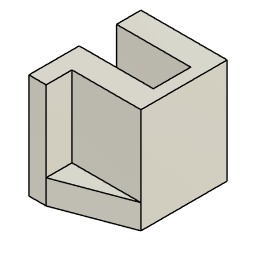
colour_sensor_servo_seat_bottom (Autodesk Fusion 360 design; units mm, degrees)
part number: 2025-09-29-11-37-15-270
part number: 2025-09-29-11-38-54-172
Autodesk Fusion 360 part; units mm, degrees
sketch "Colour Sensor Servo Seat Outline" plane through (0, 0, 0) normal (0, 0, 1) x (1, 0, 0) in component "Colour Sensor Servo Seat Bottom"
  line L0 (0, 0) -> (54.5, 0)
  line L1 (54.5, 0) -> (54.5, 39)
  line L2 (54.5, 39) -> (0, 39)
  line L3 (0, 39) -> (0, 0)
  dimension "d1" = 39
  dimension "d2" = 54.5
  constraint horizontal L0
  constraint vertical L1
  constraint horizontal L2
  constraint vertical L3
  constraint coincident L0.start L3.end
  measures "d1" distance of L0.end L1.end
  measures "d2" distance of L0.start L0.end
extrude "Extrude1" add sketch "Colour Sensor Servo Seat Outline" along normal blind 30 in component "Colour Sensor Servo Seat Bottom"
sketch "Colour Sensor Servo Hole" plane through (0, 0, 30) normal (0, 0, 1) x (-1, 0, 0) in component "Colour Sensor Servo Seat Bottom"
  line L0 (0, -39) -> (0, 0)
  line L1 (0, 0) -> (-54.5, 0)
  line L2 (-54.5, 0) -> (-54.5, -39)
  line L3 (-54.5, -39) -> (0, -39)
  line L4 (-54.5, -8.5) -> (-18, -8.5)
  line L5 (-18, -8.5) -> (-18, -21.5)
  line L6 (-18, -21.5) -> (-54.5, -21.5)
  line L7 (-54.5, -21.5) -> (-54.5, -8.5)
  line L8 (-54.5, 0) -> (-18, 0)
  line L9 (-18, 0) -> (-18, -30)
  line L10 (-18, -30) -> (-54.5, -30)
  line L11 (-54.5, -30) -> (-54.5, 0)
  line L12 (-54.5, -21.5) -> (-49.8, -21.5)
  line L13 (-49.8, -21.5) -> (-49.8, -8.5)
  line L14 (-49.8, -8.5) -> (-54.5, -8.5)
  line L15 (-54.5, -8.5) -> (-54.5, -21.5)
  point P0 (-54.5, -21.5)
  point P1 (-54.5, -30)
  dimension "d6" = 13
  dimension "d8" = 36.5
  dimension "d9" = 30
  dimension "d10" = 8.5
  dimension "d11" = 8.5
  dimension "d12" = 4.7
  constraint horizontal L4
  constraint vertical L5
  constraint horizontal L6
  constraint vertical L7
  constraint coincident L2 L4.start
  constraint horizontal L8
  constraint vertical L9
  constraint horizontal L10
  constraint vertical L11
  constraint coincident L1.end L2.start
  constraint collinear L5 L9
  constraint coincident P0 L6.end
  constraint coincident P1 L10.end
  constraint horizontal L12
  constraint vertical L13
  constraint horizontal L14
  constraint vertical L15
  constraint coincident L4 L13.end
  measures "d6" distance of L4.start P0
  measures "d8" distance of L4.start L4.end
  measures "d9" distance of L1.end P1
  measures "d10" distance of L6 L10
  measures "d11" distance of L4 L8
  measures "d12" distance of L11 L13
extrude "Extrude2" cut sketch "Colour Sensor Servo Hole" against normal blind 5 contours L2 L4 L6 L7 L11 L12 L13 L14 L15 in component "Colour Sensor Servo Seat Bottom"
extrude "Extrude3" cut sketch "Colour Sensor Servo Hole" against normal blind 25.82 contours L4 L5 L6 L9 L13 in component "Colour Sensor Servo Seat Bottom"
chamfer "Chamfer1" distance 24 distance2 9 1 edges at (27.25, 39, 0) measured on face at (36.3333, 39, 20) in component "Colour Sensor Servo Seat Bottom"
sketch "Front Ribs" plane through (0, 39, 0) normal (0, 1, 0) x (-1, 0, 0) in component "Colour Sensor Servo Seat Bottom"
  line L0 (-54.5, 24) -> (0, 24)
  line L1 (0, 24) -> (0, 30)
  line L2 (0, 30) -> (-54.5, 30)
  line L3 (-54.5, 30) -> (-54.5, 24)
  line L4 (0, 0) -> (0, 24)
  line L5 (0, 24) -> (-54.5, 24)
  line L6 (-54.5, 24) -> (-54.5, 0)
  line L7 (-54.5, 0) -> (0, 0)
  line L8 (-46, 24) -> (-18, 24)
  line L9 (-18, 24) -> (-18, 0)
  line L10 (-18, 0) -> (-46, 0)
  line L11 (-46, 0) -> (-46, 24)
  line L12 (-18, 24) -> (-9.5, 24)
  line L13 (-9.5, 24) -> (-9.5, 0)
  line L14 (-9.5, 0) -> (-18, 0)
  line L15 (-18, 0) -> (-18, 24)
  dimension "d26" = 8.5
  dimension "d31" = 8.5
  dimension "d39" = 9.5
  constraint horizontal L8
  constraint vertical L9
  constraint horizontal L10
  constraint vertical L11
  constraint coincident L7 L9.end
  constraint coincident L0 L8.start
  constraint horizontal L12
  constraint vertical L13
  constraint horizontal L14
  constraint vertical L15
  constraint coincident L7 L13.end
  measures "d26" distance of L6 L11
  measures "d31" distance of L13 L15
  measures "d39" distance of L4 L13
extrude "Extrude4" cut sketch "Front Ribs" against normal blind 9 contours L0 L5 L7 L8 L9 L10 L11 L15 | L0 L4 L5 L7 L13 in component "Colour Sensor Servo Seat Bottom"
chamfer "Chamfer2" distance 24 distance2 9.5 1 edges at (0, 15, 0) measured on face at (0, 10, 18) in component "Colour Sensor Servo Seat Bottom"
sketch "Side Ribs" plane through (0, 0, 0) normal (-1, 0, 0) x (0, -1, 0) in component "Colour Sensor Servo Seat Bottom"
  line L0 (-30, 24) -> (0, 24)
  line L1 (0, 24) -> (0, 30)
  line L2 (0, 30) -> (-39, 30)
  line L3 (-39, 30) -> (-39, 24)
  line L4 (-39, 24) -> (-30, 24)
  line L5 (0, 0) -> (0, 24)
  line L6 (0, 24) -> (-30, 24)
  line L7 (-30, 24) -> (-30, 0)
  line L8 (-30, 0) -> (0, 0)
  line L9 (-21.5, 24) -> (-8.5, 24)
  line L10 (-8.5, 24) -> (-8.5, 0)
  line L11 (-8.5, 0) -> (-21.5, 0)
  line L12 (-21.5, 0) -> (-21.5, 24)
  dimension "d33" = 8.5
  dimension "d34" = 8.5
  constraint horizontal L9
  constraint vertical L10
  constraint horizontal L11
  constraint vertical L12
  constraint coincident L8 L10.end
  constraint coincident L0 L9.start
  measures "d33" distance of L7 L12
  measures "d34" distance of L5 L10
extrude "Extrude6" cut sketch "Side Ribs" against normal blind 9.5 contours L0 L6 L8 L9 L10 L11 L12 in component "Colour Sensor Servo Seat Bottom"
chamfer "Chamfer3" distance 9.5 distance2 9 1 edges at (0, 39, 27) measured on face at (24.1667, 39, 28) in component "Colour Sensor Servo Seat Bottom"
sketch "Servo Cable Hole" plane through (9.5, 0, 0) normal (-1, 0, 0) x (0, -1, 0) in component "Colour Sensor Servo Seat Bottom"
  line L0 (-21.5, 0) -> (-8.5, 0)
  line L1 (-8.5, 0) -> (-8.5, 24)
  line L2 (-8.5, 24) -> (-21.5, 24)
  line L3 (-21.5, 24) -> (-21.5, 0)
  line L4 (-21.5, 0) -> (-21.5, 24)
  line L5 (-21.5, 24) -> (-30, 24)
  line L6 (-30, 24) -> (-30, 0)
  line L7 (-30, 0) -> (-21.5, 0)
  line L8 (-8.5, 24) -> (-8.5, 0)
  line L9 (-8.5, 0) -> (0, 0)
  line L10 (0, 0) -> (0, 24)
  line L11 (0, 24) -> (-8.5, 24)
  line L12 (-21.5, 14.18) -> (-8.5, 14.18)
  line L13 (-8.5, 14.18) -> (-8.5, 4.18)
  line L14 (-8.5, 4.18) -> (-21.5, 4.18)
  line L15 (-21.5, 4.18) -> (-21.5, 14.18)
  dimension "d40" = 10
  dimension "d41" = 4.18
  constraint horizontal L12
  constraint vertical L13
  constraint horizontal L14
  constraint vertical L15
  constraint coincident L4 L12.start
  measures "d40" distance of L12.start L14.end
  measures "d41" distance of L0 L14
extrude "Extrude7" cut sketch "Servo Cable Hole" against normal blind 8.5 contours L1 L3 L4 L8 L12 L13 L14 L15 in component "Colour Sensor Servo Seat Bottom"
sketch "Top Segment" plane through (0, 0, 0) normal (0, -1, 0) x (1, 0, 0)
  line L0 (6, 45) -> (0, 45)
  line L1 (0, 45) -> (0, 0)
  line L2 (0, 0) -> (6, 0)
  line L3 (6, 0) -> (6, 8.5)
  line L4 (6, 8.5) -> (6, 36.5)
  line L5 (6, 36.5) -> (6, 45)
  line L6 (30, 8.5) -> (6, 8.5)
  line L7 (6, 8.5) -> (6, 0)
  line L8 (6, 0) -> (30, 0)
  line L9 (30, 0) -> (30, 8.5)
  line L10 (0, 54.5) -> (0, 45)
  line L11 (0, 45) -> (6, 45)
  line L12 (6, 45) -> (6, 54.5)
  line L13 (6, 54.5) -> (0, 54.5)
  line L14 (30, 45) -> (6, 54.5)
  line L15 (6, 54.5) -> (6, 45)
  line L16 (6, 45) -> (30, 45)
  line L17 (6, 36.5) -> (30, 36.5)
  line L18 (30, 36.5) -> (30, 45)
  line L19 (30, 45) -> (6, 45)
  line L20 (6, 45) -> (6, 36.5)
  line L21 (30, 8.5) -> (30, 36.5)
  line L22 (30, 36.5) -> (6, 36.5)
  line L23 (6, 36.5) -> (6, 8.5)
  line L24 (6, 8.5) -> (30, 8.5)
  line L25 (0, 54.5) -> (30, 54.5)
  line L26 (30, 54.5) -> (30, 36.5)
  line L27 (30, 36.5) -> (0, 36.5)
  line L28 (0, 36.5) -> (0, 54.5)
  constraint horizontal L25
  constraint vertical L26
  constraint horizontal L27
  constraint vertical L28
  constraint coincident L17.end L18.start
  constraint coincident L10.start L13.end
extrude "Extrude8" cut sketch "Top Segment" against normal blind 39 contours L0 L1 L5 L11 L20 L27 L28 | L5 L16 L17 L18 L19 L20 L22 L26 L27 | L0 L10 L11 L12 L13 L15 L25 L28 | L12 L14 L15 L16 L19 | L14 L25 L26 sketch seen with x (0, 0, -1) y (0, -1, 0) z (-1, 0, 0) at (54.5, 39, 30) in component "Colour Sensor Servo Seat Bottom"
component "Colour Sensor Servo Seat Bottom" placed x (0, 0, -1) y (0, -1, 0) z (-1, 0, 0) at (30, 39, 54.5)
equation "d2 = servo_seat_width"
equation "d3 = servo_seat_height"
equation "servo_seat_height = 30 mm" comment "The height of the Colour Sensor Servo Seat component."
equation "d6 = servo_hole_width"
equation "servo_hole_width = 13 mm" comment "The width of the hole for the Colour Sensor Servo to sit in."
equation "d10 = ( 30 mm - servo_hole_width ) / 2"
equation "d13 = -servo_arm_support_depth"
equation "servo_arm_support_depth = 5 mm" comment "The depth to extrude to create the arm support for the Colour Sensor Servo."
equation "servo_hole_depth = 25.82 mm" comment "The depth to extrude to create the hole for the Colour Sensor Servo to sit in."
equation "d17 = -servo_hole_depth"
equation "d19 = servo_seat_height - top_support_thickness"
equation "d20 = 17.50 mm - 8.50 mm"
equation "top_support_thickness = 6 mm" comment "The thickness of the top supports that will go underneath the Colour Detection Mechanism Platform."
equation "d22 = -( 17.50 mm - 8.50 mm )"
equation "rib_thickness = 8.5 mm" comment "The thickness of the support ribs."
equation "d26 = rib_thickness"
equation "d27 = servo_seat_height - top_support_thickness"
equation "d28 = servo_seat_width - 36.50 mm - 8.5 mm"
equation "d31 = rib_thickness"
equation "servo_seat_width = 36.50 mm + 18 mm" comment "The width of the Colour Sensor Servo Seat component."
equation "d33 = rib_thickness"
equation "d34 = rib_thickness"
equation "d35 = -( servo_seat_width - 36.50 mm - 8.5 mm )"
equation "d37 = ( servo_seat_width - 36.50 mm - 8.5 mm )"
equation "d39 = ( servo_seat_width - 36.50 mm - 8.5 mm )"
equation "d41 = servo_seat_height - servo_hole_depth"
equation "d42 = -rib_thickness"
named bodies: "Colour Sensor Servo Seat Bottom"
